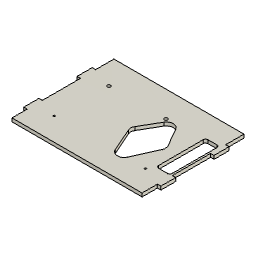
Display Plate (Autodesk Fusion 360 design; units mm, degrees)
Autodesk Fusion 360 part; units mm, degrees
sketch "Sketch1" plane through (0, 0, 0) normal (0, 0, 1) x (1, 0, 0)
  line L0 (90, -67) -> (-90, -67)
  line L1 (-90, -67) -> (-90, 67)
  line L2 (-90, 67) -> (90, 67)
  line L3 (90, 67) -> (90, -67)
  line L4 (90, -67) -> (-90, 67) construction
  line L5 (-90, -67) -> (90, 67) construction
  line L6 (-85.5, 67) -> (-85.5, -67)
  line L7 (85.5, 67) -> (85.5, -67)
  line L8 (-85.5, -67) -> (-90, -67)
  line L9 (-90, -67) -> (-90, -47)
  line L10 (-90, -47) -> (-85.5, -47)
  line L11 (-85.5, -47) -> (-85.5, -67)
  line L12 (-85.5, -47) -> (-90, -47)
  line L13 (-90, -47) -> (-90, -27)
  line L14 (-90, -27) -> (-85.5, -27)
  line L15 (-85.5, -27) -> (-85.5, -47)
  line L16 (-85.5, -27) -> (-90, -27)
  line L17 (-90, -27) -> (-90, 23)
  line L18 (-90, 23) -> (-85.5, 23)
  line L19 (-85.5, 23) -> (-85.5, -27)
  line L20 (-85.5, 23) -> (-90, 23)
  line L21 (-90, 23) -> (-90, 43)
  line L22 (-90, 43) -> (-85.5, 43)
  line L23 (-85.5, 43) -> (-85.5, 23)
  line L24 (90, -67) -> (85.5, -67)
  line L25 (85.5, -67) -> (85.5, -47)
  line L26 (85.5, -47) -> (90, -47)
  line L27 (90, -47) -> (90, -67)
  line L28 (90, -47) -> (85.5, -47)
  line L29 (85.5, -47) -> (85.5, -27)
  line L30 (85.5, -27) -> (90, -27)
  line L31 (90, -27) -> (90, -47)
  line L32 (90, -27) -> (85.5, -27)
  line L33 (85.5, -27) -> (85.5, 23)
  line L34 (85.5, 23) -> (90, 23)
  line L35 (90, 23) -> (90, -27)
  line L36 (90, 23) -> (85.5, 23)
  line L37 (85.5, 23) -> (85.5, 43)
  line L38 (85.5, 43) -> (90, 43)
  line L39 (90, 43) -> (90, 23)
  line L40 (-90, 33) -> (90, 33) construction
  circle A0 centre (-58, 33) radius 2.15
  circle A1 centre (17, 33) radius 2.15
  line L41 (0, 67) -> (0, 33.0008) construction
  line L42 (-90, -37) -> (90, -37) construction
  circle A2 centre (-60, -37) radius 1.15
  circle A3 centre (60, -37) radius 1.15
  line L43 (80, -28) -> (68, -28)
  line L44 (65, -25) -> (65, 34)
  line L45 (68, 37) -> (80, 37)
  line L46 (83, 34) -> (83, -25)
  line L47 (83, -28) -> (65, 37) construction
  line L48 (65, -28) -> (83, 37) construction
  arc A4 (68, 37) -> (65, 34) centre (68, 34) ccw
  arc A5 (83, 34) -> (80, 37) centre (80, 34) ccw
  arc A6 (80, -28) -> (83, -25) centre (80, -25) ccw
  arc A7 (65, -25) -> (68, -28) centre (68, -25) ccw
  circle A8 centre (27, 23.5) radius 9
  line L49 (27, 67) -> (27, -67) construction
  circle A9 centre (27, -32) radius 9
  line L50 (27, -24.0416) -> (2.9584, 0)
  line L51 (2.9584, 0) -> (27, 24.0416)
  line L52 (27, 24.0416) -> (51.0416, 0)
  line L53 (51.0416, 0) -> (27, -24.0416)
  line L54 (27, -24.0416) -> (27, 24.0416) construction
  line L55 (2.9584, 0) -> (51.0416, 0) construction
  line L56 (48.7377, 3.9705) -> (34.7844, 28.017)
  line L57 (5.2623, 3.9705) -> (19.2156, 28.017)
  line L58 (4.8198, -4.1961) -> (18.7732, -35.6496)
  line L59 (49.1802, -4.1961) -> (35.2268, -35.6496)
  arc A10 (5.2623, 3.9705) -> (4.8198, -4.1961) centre (13.0467, -0.5465) ccw
  arc A11 (49.1802, -4.1961) -> (48.7377, 3.9705) centre (40.9533, -0.5465) ccw
  point P0 (74, 4.5)
  point P1 (27, 0)
  dimension "d1" = 180
  dimension "d2" = 134
  dimension "d3" = 4.5
  dimension "d4" = 4.5
  dimension "d5" = 20
  dimension "d6" = 20
  dimension "d7" = 50
  dimension "d8" = 20
  dimension "d9" = 20
  dimension "d10" = 20
  dimension "d11" = 50
  dimension "d12" = 20
  dimension "d13" = 4.3
  dimension "d14" = 4.3
  dimension "d15" = 75
  dimension "d16" = 17
  dimension "d17" = 70
  dimension "d18" = 2.3
  dimension "d19" = 2.3
  dimension "d20" = 60
  dimension "d21" = 60
  dimension "d22" = 33
  dimension "d23" = 18
  dimension "d24" = 65
  dimension "d25" = 5
  dimension "d26" = 3
  dimension "d27" = 3
  dimension "d28" = 3
  dimension "d29" = 3
  dimension "d35" = 18
  dimension "d36" = 27
  dimension "d37" = 23.5
  dimension "d38" = 18
  dimension "d39" = 34
  dimension "d40" = 34
  dimension "d41" = 9
  dimension "d42" = 9
  dimension "d57" = 32
  dimension "d58" = 30
  constraint horizontal L0
  constraint perpendicular L0 L1
  constraint parallel L0 L2
  constraint parallel L1 L3
  constraint coincident L4 origin
  constraint coincident L5 origin
  constraint coincident L2 L6.start
  constraint coincident L0 L6.end
  constraint perpendicular L0 L6
  constraint coincident L2 L7.start
  constraint coincident L0 L7.end
  constraint perpendicular L0 L7
  constraint horizontal L8
  constraint vertical L9
  constraint horizontal L10
  constraint vertical L11
  constraint horizontal L12
  constraint vertical L13
  constraint horizontal L14
  constraint vertical L15
  constraint horizontal L16
  constraint vertical L17
  constraint horizontal L18
  constraint vertical L19
  constraint horizontal L20
  constraint vertical L21
  constraint horizontal L22
  constraint vertical L23
  constraint horizontal L24
  constraint vertical L25
  constraint horizontal L26
  constraint vertical L27
  constraint horizontal L28
  constraint vertical L29
  constraint horizontal L30
  constraint vertical L31
  constraint horizontal L32
  constraint vertical L33
  constraint horizontal L34
  constraint vertical L35
  constraint horizontal L36
  constraint vertical L37
  constraint horizontal L38
  constraint vertical L39
  constraint coincident L1 L40.start
  constraint coincident L3 L40.end
  constraint perpendicular L3 L40
  constraint coincident L40 A0.centre
  constraint coincident L40 A1.centre
  constraint midpoint L2 L41.start
  constraint perpendicular L40 L41
  constraint coincident L1 L42.start
  constraint coincident L13 L42.start
  constraint coincident L31 L42.end
  constraint perpendicular L31 L42
  constraint coincident L42 A2.centre
  constraint coincident L42 A3.centre
  constraint horizontal L43
  constraint perpendicular L43 L44
  constraint parallel L43 L45
  constraint parallel L44 L46
  constraint coincident L47.end L44
  constraint coincident L47.end L45
  constraint tangent L44 A4
  constraint tangent L45 A4
  constraint coincident L48.end L46
  constraint coincident L48.end L45
  constraint tangent L46 A5
  constraint tangent L45 A5
  constraint coincident L47.start L46
  constraint coincident L47.start L43
  constraint tangent L46 A6
  constraint tangent L43 A6
  constraint coincident L48.start L43
  constraint coincident L48.start L44
  constraint tangent L43 A7
  constraint tangent L44 A7
  constraint coincident L2 L49.start
  constraint coincident L0 L49.end
  constraint perpendicular L0 L49
  constraint coincident A8.centre L49
  constraint coincident L49 A9.centre
  constraint perpendicular L50 L51
  constraint parallel L50 L52
  constraint parallel L51 L53
  constraint coincident L54 P1
  constraint coincident L55 P1
  constraint midpoint L49 P1
  constraint coincident A8 L56.end
  constraint tangent A8 L56
  constraint coincident A8 L57.end
  constraint tangent A8 L57
  constraint coincident A9 L58.end
  constraint tangent A9 L58
  constraint coincident A9 L59.end
  constraint tangent A9 L59
  constraint coincident L50.end L58
  constraint coincident L50.end L57
  constraint tangent L58 A10
  constraint tangent L57 A10
  constraint coincident L52.end L56
  constraint coincident L52.end L59
  constraint tangent L56 A11
  constraint tangent L59 A11
  constraint coincident L49 L51.end
  constraint midpoint L48 P0
  measures "d1" distance of L1.end L2.end
  measures "d2" distance of L0.end L1.end
  measures "d3" distance of L3 L7
  measures "d4" distance of L1 L6
  measures "d5" distance of L6.end L10.end
  measures "d6" distance of L10.end L14.end
  measures "d7" distance of L14.end L18.end
  measures "d8" distance of L18.end L22.end
  measures "d9" distance of L0.start L26.end
  measures "d10" distance of L26.end L30.end
  measures "d11" distance of L30.end L34.end
  measures "d12" distance of L34.end L38.end
  measures "d13" diameter of A0
  measures "d14" diameter of A1
  measures "d15" distance of A0.centre A1.centre
  measures "d16" distance of A1.centre L41
  measures "d17" distance of L40 L42
  measures "d18" diameter of A2
  measures "d19" diameter of A3
  measures "d20" distance of L41 A3.centre
  measures "d21" distance of L41 A2.centre
  measures "d22" distance of origin L40
  measures "d23" distance of L47.end L48.end
  measures "d24" distance of L48.start L47.end
  measures "d25" distance of A3.centre L44
  measures "d26" radius of A4
  measures "d27" radius of A5
  measures "d28" radius of A6
  measures "d29" radius of A7
  measures "d35" diameter of A8
  measures "d36" distance of L41 L49
  measures "d37" vertical distance of origin A8.centre
  measures "d38" diameter of A9
  measures "d39" distance of L51.end L52.end
  measures "d40" distance of L50.end L51.end
  measures "d41" radius of A10
  measures "d42" radius of A11
  measures "d57" distance of A9.centre L55
  measures "d58" distance of L2 L45
extrude "Extrude1" add sketch "Sketch1" along normal blind 4.5 contours L0 L2 L6 L7 L11 L15 L19 L23 L25 L29 L33 L37 | L3 L7 L26 L28 L29 L30 L31 L32 | L1 L6 L10 L12 L13 L14 L15 L16 | L3 L7 L34 L36 L37 L38 L39 | L1 L6 L18 L20 L21 L22 L23 | L52 L53 A11 | L50 L51 A10
move_face "OffsetFaces1" offset -0.1 4 faces at (87, 23, 1.5) (87, -47, 1.5) (-88.5, 23, 1.5) (-88.5, -47, 1.5)
move_face "OffsetFaces2" offset -0.1 4 faces at (87, -27, 1.5) (87, 43, 1.5) (-88.5, -27, 1.5) (-88.5, 43, 1.5)
